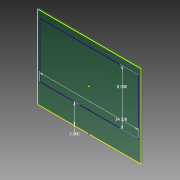
# Autodesk Inventor part: glass-print-bed
Saved by Autodesk Inventor 2015 (Build 190159000, 159)
## iProperties
Created: 2014-10-22
Part Number: glass-print-bed
Material: Generic
Document SubType Name: Modeling
Designer: caleb
Density: 1 g/cm^3
Appearance: Clear - Green 1
Author: caleb
Autodesk Inventor part; units mm, degrees
ref_plane "YZ Plane" through (0, 0, 0) normal (1, 0, 0) x (0, 1, 0)
ref_plane "XZ Plane" through (0, 0, 0) normal (0, 1, 0) x (-1, 0, 0)
ref_plane "XY Plane" through (0, 0, 0) normal (0, 0, 1) x (1, 0, 0)
sketch "Sketch1" plane through (0, 0, 0) normal (0, 0, 1) x (1, 0, 0)
  line L0 (-190.5, -152.4) -> (190.5, -152.4)
  line L1 (190.5, -152.4) -> (190.5, 152.4)
  line L2 (190.5, 152.4) -> (-190.5, 152.4)
  line L3 (-190.5, 152.4) -> (-190.5, -152.4)
  line L4 (-190.5, -152.4) -> (190.5, 152.4) construction
  line L5 (190.5, -152.4) -> (-190.5, 152.4) construction
  point P0 (0, 0)
  dimension "d0" = 304.8
  dimension "d1" = 381
  constraints: 12 end point, 2 midpoint, 2 parallel, 1 horizontal, 1 perpendicular
  measures "d0" distance of L0.end L1.end
  measures "d1" distance of L0.start L0.end
extrude "Extrusion1" add sketch "Sketch1" along normal blind 6.35
sketch "Sketch2" plane through (0, 0, 6.35) normal (0, 0, 1) x (1, 0, 0)
  line L0 (-182.5625, -76.2) -> (182.5625, -76.2)
  line L1 (182.5625, -76.2) -> (182.5625, 127)
  line L2 (182.5625, 127) -> (-182.5625, 127)
  line L3 (-182.5625, 127) -> (-182.5625, -76.2)
  line L4 (-190.5, -152.4) -> (190.5, -152.4) projected
  line L5 (190.5, -152.4) -> (190.5, 152.4) projected
  line L6 (190.5, 152.4) -> (-190.5, 152.4) projected
  line L7 (-190.5, 152.4) -> (-190.5, -152.4) projected
  point P0 (0, 0)
  point P1 (0, -76.2)
  point P2 (0, -152.4)
  dimension "d4" = 76.2
  dimension "d5" = 365.125
  dimension "d6" = 203.2
  constraints: 8 end point, 2 midpoint, 2 parallel, 1 horizontal, 1 perpendicular, 1 vertical alignment
  measures "d4" distance between parallel lines of L4 L0
  measures "d5" distance of L0.start L0.end
  measures "d6" distance of L0.end L1.end
body "Solid1"
